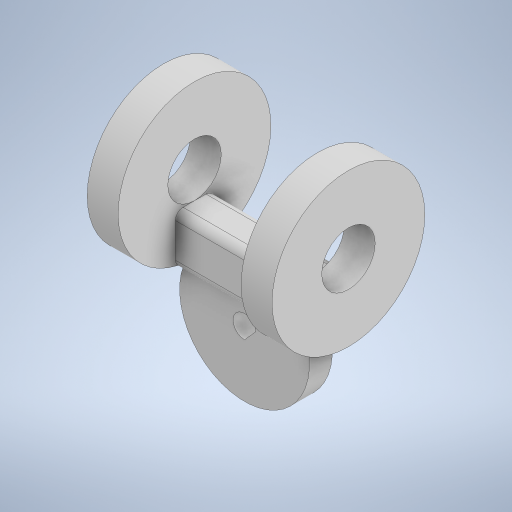
# Autodesk Inventor part: KnuclePart
Saved by Autodesk Inventor 2024 (Build 280153000, 153)
## iProperties
Created: 2024-03-22
Part Number: KnuclePart
Material: Generic
Document SubType Name: Modeling
Designer: Wojtek
Density: 1 g/cm^3
Appearance: Default
Author: Wojtek
Autodesk Inventor part; units mm, degrees
ref_plane "YZ Plane" through (0, 0, 0) normal (1, 0, 0) x (0, 1, 0)
ref_plane "XZ Plane" through (0, 0, 0) normal (0, 1, 0) x (-1, 0, 0)
ref_plane "XY Plane" through (0, 0, 0) normal (0, 0, 1) x (1, 0, 0)
sketch "Sketch1" plane through (0, 0, 0) normal (1, 0, 0) x (0, 1, 0)
  circle A0 centre (0, 0) radius 10
  circle A1 centre (0, 0) radius 3.5
  dimension "d0" = 20
  dimension "d1" = 7
  constraints: 2 centre point, 2 coincident
  measures "d0" diameter of A0
  measures "d1" diameter of A1
extrude "Extrusion1" add sketch "Sketch1" along normal mid plane 24.2
extrude "Extrusion2" cut sketch "Sketch1" along normal mid plane 16.1
sketch "Sketch2" plane through (0, 0, 0) normal (0, 0, 1) x (1, 0, 0)
  line L0 (-8.05, -3.5) -> (-8.05, 3.5) projected
  line L1 (8.05, -10) -> (8.05, 10) projected
  line L2 (-8.05, -3.5) -> (8.05, -3.5)
  line L3 (8.05, -3.5) -> (8.05, -10)
  line L4 (8.05, -10) -> (-8.05, -10)
  line L5 (-8.05, -10) -> (-8.05, -3.5)
  circle A0 centre (0, -13) radius 8.5
  point P0 (0, 0)
  point P1 (0, -10)
  point P2 (-7.953, -10)
  point P3 (7.953, -10)
  dimension "d9" = 17
  dimension "d10" = 3
  dimension "d11" = 13
  dimension "d19" = 6.5
  constraints: 8 end point, 2 parallel, 1 centre point, 1 horizontal, 1 midpoint, 1 perpendicular
  measures "d9" diameter of A0
  measures "d10" distance of A0.centre point (0, -10)
  measures "d11" distance of point (0, 0) A0.centre
  measures "d19" distance of L4.end L0.start
extrude "Extrusion3" add sketch "Sketch2" along normal mid plane 5 contours L4 A0 L5 L2 L1 | L4 A0 picked at (2.3341, -9.3938)
fillet "Fillet1" radius 1 4 edges at (0, -3.5, 2.5) (0, -3.5, -2.5) (0, -10, 2.5) (0, -10, -2.5)
extrude "Extrusion4" add sketch "Sketch2" along normal mid plane 3 contours A0 L4 picked at (-0.095, -17.4274)
sketch "Sketch3" plane through (0, 0, 1.5) normal (0, 0, 1) x (1, 0, 0)
  arc A0 (-7.953, -10) -> (7.953, -10) centre (0, -13) ccw projected
  circle A1 centre (0, -13) radius 1.5
  line L0 (0, -14.5) -> (1.4907, -12.8334)
  line L1 (-7.953, -10) -> (7.953, -10) projected
  point P0 (0, 0)
  dimension "d14" = 3
  dimension "d15" = 2.236
  dimension "d16" = 4.5
  constraints: 2 coincident, 2 end point, 2 point on circle, 1 centre point
  measures "d14" diameter of A1
  measures "d15" distance of L0.start L0.end
  measures "d16" distance from line of L1 L0.start
extrude "Extrusion5" cut sketch "Sketch3" against normal blind 3 contours L0 A1 picked at (0.0848, -13.7277)
body "Solid1"
